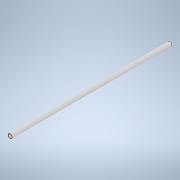
# Autodesk Inventor part: perpendicular horizontal bar
Saved by Autodesk Inventor 2021 (Build 250183000, 183)
## iProperties
Created: 2020-07-11
Part Number: perpendicular horizontal bar
Material: Generic
Document SubType Name: Modeling
Designer: Shannon
Density: 1 g/cm^3
Appearance: Default
Author: Shannon
Autodesk Inventor part; units mm, degrees
ref_plane "YZ Plane" through (0, 0, 0) normal (1, 0, 0) x (0, 1, 0)
ref_plane "XZ Plane" through (0, 0, 0) normal (0, 1, 0) x (-1, 0, 0)
ref_plane "XY Plane" through (0, 0, 0) normal (0, 0, 1) x (1, 0, 0)
sketch "Sketch1" plane through (0, 0, 0) normal (0, 0, 1) x (1, 0, 0)
  circle A0 centre (0, 0) radius 6.35
  dimension "d0" = 12.7
  constraints: 1 centre point, 1 coincident
  measures "d0" diameter of A0
extrude "Extrusion1" add sketch "Sketch1" along normal blind 474.98
sketch "Sketch2" plane through (0, 0, 474.98) normal (0, 0, 1) x (1, 0, 0)
  circle A0 centre (0, 0) radius 5.334
  dimension "d3" = 10.668
  constraints: 1 centre point, 1 coincident
  measures "d3" diameter of A0
extrude "Extrusion2" cut sketch "Sketch2" against normal blind 660.4
body "Solid1"
